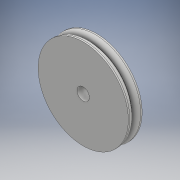
# Autodesk Inventor part: Raket_Hjul
Saved by Autodesk Inventor 2018 (Build 220112000, 112)
## iProperties
Created: 2017-08-14
Part Number: Raket_Hjul
Material: Generic
Document SubType Name: Modeling
Designer: andre
Density: 1 g/cm^3
Appearance: Default
Author: andre
## iProperties of the stored document Raket_Hjul_3DPrint.ipt
Created: 2017-08-14
Part Number: Raket_Hjul_3DPrint
Material: Generic
Document SubType Name: Modeling
Designer: andre
Density: 1 g/cm^3
Appearance: Default
Author: andre
Autodesk Inventor part; units mm, degrees
ref_plane "YZ Plane" through (0, 0, 0) normal (1, 0, 0) x (0, 1, 0)
ref_plane "XZ Plane" through (0, 0, 0) normal (0, 1, 0) x (-1, 0, 0)
ref_plane "XY Plane" through (0, 0, 0) normal (0, 0, 1) x (1, 0, 0)
sketch "Sketch1" plane through (0, 0, 0) normal (0, 1, 0) x (-1, 0, 0)
  circle A0 centre (0, 0) radius 15
  circle A1 centre (0, 0) radius 2.05
  dimension "d0" = 30
  dimension "d1" = 4.1
  constraints: 2 centre point, 2 coincident
  measures "d0" diameter of A0
  measures "d1" diameter of A1
extrude "Extrusion1" add sketch "Sketch1" along normal blind 2
sketch "Sketch2" plane through (0, 2, 0) normal (0, 1, 0) x (1, 0, 0)
  circle A0 centre (0, 0) radius 13.5
  circle A1 centre (0, 0) radius 2.05
  dimension "d4" = 27
  constraints: 2 centre point, 1 coincident
  measures "d4" diameter of A0
extrude "Extrusion2" add sketch "Sketch2" along normal blind 0.5
sketch "Sketch3" plane through (0, 2.5, 0) normal (0, 1, 0) x (1, 0, 0)
  circle A0 centre (0, 0) radius 15.1009
  circle A1 centre (0, 0) radius 2.05
  constraints: 2 centre point, 1 coincident
extrude "Extrusion3" add sketch "Sketch3" along normal blind 2
fillet "Fillet1" radius 1.5 2 edges at (15, 2, 0) (-15.1009, 2.5, 0)
body "Solid1"
